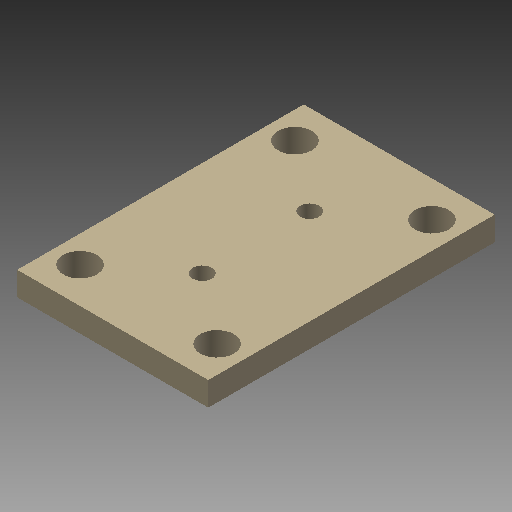
# Autodesk Inventor part: Shield_1
Saved by Autodesk Inventor 2018 (Build 220112000, 112)
## iProperties
Created: 2015-02-10
Part Number: Shield_1
Material: Generic
Document SubType Name: Modeling
Designer: Pascal
Density: 1 g/cm^3
Appearance: Beige
Author: Pascal
Autodesk Inventor part; units mm, degrees
ref_plane "YZ Plane" through (0, 0, 0) normal (1, 0, 0) x (0, 1, 0)
ref_plane "XZ Plane" through (0, 0, 0) normal (0, 1, 0) x (-1, 0, 0)
ref_plane "XY Plane" through (0, 0, 0) normal (0, 0, 1) x (1, 0, 0)
sketch "Sketch1" plane through (0, 0, 0) normal (0, 1, 0) x (-1, 0, 0)
  line L0 (13.2677, 19.6408) -> (-12.1323, 19.6408)
  line L1 (-12.1323, 19.6408) -> (-12.1323, -18.4592)
  line L2 (-12.1323, -18.4592) -> (13.2677, -18.4592)
  line L3 (13.2677, -18.4592) -> (13.2677, 19.6408)
  point P0 (0, 0)
  dimension "d0" = 25.4
  dimension "d1" = 38.1
  constraints: 8 end point, 2 parallel, 1 horizontal, 1 perpendicular
  measures "d0" distance of L1.end L2.end
  measures "d1" distance of L2.end L0.start
extrude "Extrusion1" add sketch "Sketch1" along normal blind 3.175
hole "Hole1" at (-9.6799, 3.175, 14.8783) direction (0, -1, 0) diameter 4.4958 depth 3.175 clearance for "Flat Head Machine Screw (82)" size "#8" standard "Ansi Unified Screw Threads"
hole "Hole2" at (8.5446, 3.175, 14.8783) direction (0, -1, 0) diameter 4.4958 depth 3.175 clearance for "Flat Head Machine Screw (82)" size "#8" standard "Ansi Unified Screw Threads"
hole "Hole3" at (-9.6799, 3.175, -13.6967) direction (0, -1, 0) diameter 4.4958 depth 3.175 clearance for "Flat Head Machine Screw (82)" size "#8" standard "Ansi Unified Screw Threads"
hole "Hole4" at (8.5446, 3.175, -13.6967) direction (0, -1, 0) diameter 4.4958 depth 3.175 clearance for "Flat Head Machine Screw (82)" size "#8" standard "Ansi Unified Screw Threads"
hole "Hole5" at (-0.5677, 3.175, -6.5466) direction (0, -1, 0) diameter 2.54 depth 3.175
hole "Hole6" at (-0.5677, 3.175, 7.7345) direction (0, -1, 0) diameter 2.54 depth 3.175
body "Solid1"
